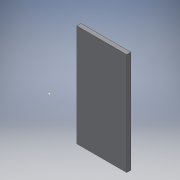
# Autodesk Inventor part: XMotorMount
Saved by Autodesk Inventor 2019 (Build 230136000, 136)
## iProperties
Created: 2018-10-14
Part Number: XMotorMount
Material: Generic
Document SubType Name: Modeling
Designer: LillaHunden
Density: 1 g/cm^3
Appearance: Default
Author: LillaHunden
Autodesk Inventor part; units mm, degrees
ref_plane "YZ Plane" through (0, 0, 0) normal (1, 0, 0) x (0, 1, 0)
ref_plane "XZ Plane" through (0, 0, 0) normal (0, 1, 0) x (-1, 0, 0)
ref_plane "XY Plane" through (0, 0, 0) normal (0, 0, 1) x (1, 0, 0)
sketch "Sketch1" plane through (0, 0, 0) normal (0, 0, 1) x (1, 0, 0)
  line L0 (112.0815, -42.6698) -> (40.0716, -42.6698)
  line L1 (40.0716, -42.6698) -> (40.0716, 105.1384)
  line L2 (40.0716, 105.1384) -> (112.0815, 105.1384)
  line L3 (112.0815, 105.1384) -> (112.0815, -42.6698)
  point P0 (0, 0)
  constraints: 8 end point, 2 parallel, 1 horizontal, 1 perpendicular
extrude "Extrusion1" add sketch "Sketch1" along normal blind 6
sketch "Sketch2" plane through (0, 0, 6) normal (0, 0, 1) x (1, 0, 0)
  point P0 (0, 0)
sketch "Sketch3" plane through (0, 0, 6) normal (0, 0, 1) x (1, 0, 0)
  circle A0 centre (45.9019, 18.4802) radius 3.25 construction
  circle A1 centre (55.0716, 18.4786) radius 3.25 construction
  circle A2 centre (55.0716, 11.1818) radius 3.25 construction
  circle A3 centre (45.9019, 11.1802) radius 3.25 construction
  line L0 (-13.5113, 7.3302) -> (60.0076, 7.3302) construction
  line L1 (60.0076, 7.3302) -> (60.0076, 22.3302) construction
  line L2 (-13.5113, 22.3302) -> (60.0076, 22.3302) construction
  line L3 (-13.5113, 7.3302) -> (-13.5113, 22.3302) construction
  line L4 (40.0716, 105.1384) -> (40.0716, -42.6698) projected
  line L5 (40.0716, 23.8302) -> (61.5076, 23.8302)
  line L6 (61.5076, 23.8302) -> (61.5076, 5.8302)
  line L7 (61.5076, 5.8302) -> (40.0716, 5.8302)
  line L8 (40.0716, 5.8302) -> (40.0716, 23.8302)
  point P0 (0, 0)
  dimension "d2" = 1.5
  dimension "d3" = 1.5
  dimension "d4" = 1.5
  constraints: 8 end point, 2 parallel, 1 horizontal, 1 perpendicular, 1 point on line
  measures "d2" distance between parallel lines of L0 L7
  measures "d3" distance between parallel lines of L5 L2
  measures "d4" distance between parallel lines of L6 L1
extrude "Extrusion2" cut sketch "Sketch3" against normal through all
body "Solid1"
